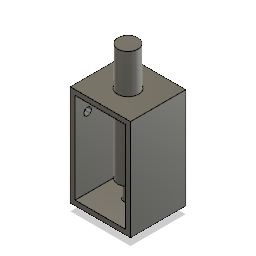
Fusion360_Solenoid_ZHO-0420S-05A4 (Autodesk Fusion 360 design; units mm, degrees)
Autodesk Fusion 360 part; units mm, degrees
sketch "スケッチ1" plane through (0, 0, 0) normal (0, 1, 0) x (1, 0, 0)
  line L0 (6, -5.5) -> (-6, -5.5)
  line L1 (-6, -5.5) -> (-6, 5.5)
  line L2 (-6, 5.5) -> (6, 5.5)
  line L3 (6, 5.5) -> (6, -5.5)
  line L4 (6, -5.5) -> (-6, 5.5) construction
  line L5 (-6, -5.5) -> (6, 5.5) construction
  dimension "d1" = 12
  dimension "d2" = 11
extrude "押し出し1" add sketch "スケッチ1" along normal blind 20 makes body 1 in component "Component'"
sketch "スケッチ2" plane through (0, 0, 5.5) normal (0, 0, 1) x (1, 0, 0)
  line L0 (-6, 0) -> (6, 0)
  line L1 (6, 0) -> (6, 20)
  line L2 (6, 20) -> (-6, 20)
  line L3 (-6, 20) -> (-6, 0)
  line L4 (-5, 1) -> (5, 1)
  line L5 (5, 1) -> (5, 19)
  line L6 (5, 19) -> (-5, 19)
  line L7 (-5, 19) -> (-5, 1)
extrude "押し出し2" cut sketch "スケッチ2" against normal blind 24 contours L4 L5 L6 L7 bodies 1 in component "Component'"
sketch "スケッチ3" plane through (0, 20, 0) normal (0, 1, 0) x (-1, 0, 0)
  line L0 (-6, -5.5) -> (6, -5.5)
  line L1 (6, -5.5) -> (6, 5.5)
  line L2 (6, 5.5) -> (-6, 5.5)
  line L3 (-6, 5.5) -> (-6, -5.5)
  circle A0 centre (0, 0) radius 2.1
  dimension "d7" = 4.2
  measures "d7" diameter of A0
extrude "押し出し3" cut sketch "スケッチ3" against normal blind 6 contours A0 bodies 1 in component "Component'"
sketch "スケッチ4" plane through (0, 1, 0) normal (0, 1, 0) x (-1, 0, 0)
  line L0 (-5, -5.5) -> (5, -5.5)
  line L1 (5, -5.5) -> (5, 5.5)
  line L2 (5, 5.5) -> (-5, 5.5)
  line L3 (-5, 5.5) -> (-5, -5.5)
  circle A0 centre (0, 0) radius 0.9
  dimension "d10" = 1.8
  measures "d10" diameter of A0
extrude "押し出し4" cut sketch "スケッチ4" against normal blind 1.5 contours A0 bodies 1 in component "Component'"
sketch "スケッチ5" plane through (0, 0, 0) normal (0, 1, 0) x (1, 0, 0)
  circle A0 centre (0, 0) radius 0.8
  dimension "d13" = 1.6
  measures "d13" diameter of A0
extrude "押し出し1'" add sketch "スケッチ5" against normal blind 3.5 separate body makes body 2 in component "Component''"
sketch "スケッチ6" plane through (0, -3.5, 0) normal (0, -1, 0) x (1, 0, 0)
  circle A0 centre (0, 0) radius 0.8
  circle A1 centre (0, 0) radius 1.5
  dimension "d16" = 3
  measures "d16" diameter of A1
extrude "押し出し2'" add sketch "スケッチ6" along normal blind 1.4 contours A0 | A1 bodies 2 in component "Component''"
move_face "面をオフセット1" offset 1 1 faces at (0.273, 0, -0.1637) on bodies 2 in component "Component''"
sketch "スケッチ7" plane through (0, 1, 0) normal (0, 1, 0) x (-1, 0, 0)
  circle A0 centre (0, 0) radius 0.8
  circle A1 centre (0, 0) radius 2
  dimension "d20" = 4
  measures "d20" diameter of A1
extrude "押し出し3'" add sketch "スケッチ7" along normal blind 23.2 contours A0 | A1 bodies 2 in component "Component''"
sketch "スケッチ8" plane through (-6, 0, 0) normal (-1, 0, 0) x (0, 0, 1)
  line L0 (-5.5, 0) -> (5.5, 0)
  line L1 (5.5, 0) -> (5.5, 20)
  line L2 (5.5, 20) -> (-5.5, 20)
  line L3 (-5.5, 20) -> (-5.5, 0)
  line L4 (-5.5, 0) -> (-3, 0) construction
  line L5 (-3, 0) -> (-3, 5) construction
  line L6 (-3, 5) -> (-5.5, 5) construction
  line L7 (-5.5, 5) -> (-5.5, 0) construction
  circle A0 centre (-3, 5) radius 0.75
  dimension "d23" = 2.5
  dimension "d24" = 5
  dimension "d25" = 1.5
  measures "d25" diameter of A0
extrude "押し出し5" cut sketch "スケッチ8" against normal blind 2 contours A0 bodies 1 in component "Component'"
sketch "スケッチ9" plane through (-6, 0, 0) normal (-1, 0, 0) x (0, 0, 1)
  circle A0 centre (-3, 5) radius 0.75
  line L0 (-5.5, 0) -> (5.5, 0)
  line L1 (5.5, 0) -> (5.5, 20)
  line L2 (5.5, 20) -> (-5.5, 20)
  line L3 (-5.5, 20) -> (-5.5, 0)
  line L4 (5.5, 0) -> (3, 0) construction
  line L5 (3, 0) -> (3, 15) construction
  line L6 (3, 15) -> (5.5, 15) construction
  line L7 (5.5, 15) -> (5.5, 0) construction
  circle A1 centre (3, 15) radius 0.75
  dimension "d28" = 15
  dimension "d29" = 2.5
  dimension "d30" = 1.5
  measures "d30" diameter of A1
extrude "押し出し6" cut sketch "スケッチ9" against normal blind 2 contours A1 bodies 1 in component "Component'"
component "Component'" placed x (1, 0, 0) y (0, 1, 0) z (0, 0, 1) at (0, 0, 0)
component "Component''" placed x (1, 0, 0) y (0, 1, 0) z (0, 0, 1) at (0, 3.5, 0)
